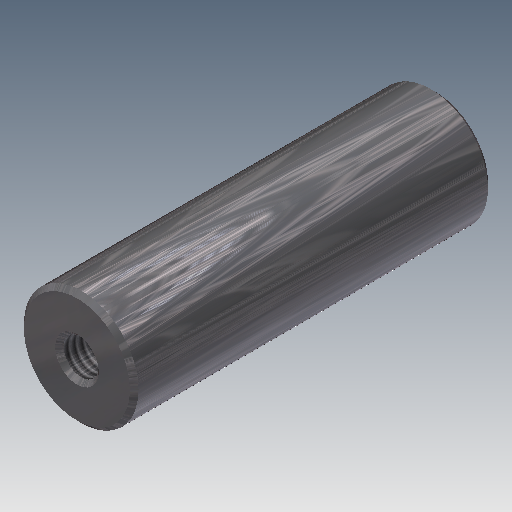
# Autodesk Inventor part: ラックギア側ベアリング軸
Saved by Autodesk Inventor 2019.4 (Build 234330000, 330)
## iProperties
Created: 2018-08-09
Part Number: ラックギア側ベアリング軸
Material: アルミニウム 2014-T4
Document SubType Name: Modeling
Designer: Owner
Density: 2.8 g/cm^3
Appearance: サテン
Mass: 3.17787 g
Surface Area: 9.00932 cm^2
Volume: 1.13495 cm^3
Author: Owner
Autodesk Inventor part; units mm, degrees
ref_plane "YZ Plane" through (0, 0, 0) normal (1, 0, 0) x (0, 1, 0)
ref_plane "XZ Plane" through (0, 0, 0) normal (0, 1, 0) x (-1, 0, 0)
ref_plane "XY Plane" through (0, 0, 0) normal (0, 0, 1) x (1, 0, 0)
sketch "スケッチ1" plane through (0, 0, 0) normal (0, 0, 1) x (1, 0, 0)
  circle A0 centre (0, 0) radius 4
  dimension "d0" = 8
  constraints: 1 centre point, 1 coincident
  measures "d0" diameter of A0
extrude "押し出し1" add sketch "スケッチ1" along normal mid plane 25
sketch "スケッチ2" plane through (0, 0, -12.5) normal (0, 0, -1) x (-1, 0, 0)
  point P0 (0, 0)
hole "穴1" at (0, 0, -12.5) direction (0, 0, 1) diameter 2.459 end through all thread size "M3x0.5" class "6H" standard "ISO Metric profile"
thread "ねじ1" size "M3x0.5" class "6H" standard "ANSI Metric M Profile" full length
chamfer "面取り1" distance 0.3 angle 45 4 edges at (0, -1.2295, -12.5) (-4, 0, -12.5) (0, -1.2295, 12.5) (-4, 0, 12.5)
